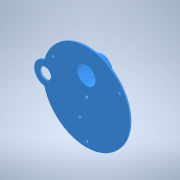
# Autodesk Inventor part: filterTop
Saved by Autodesk Inventor 2022.1 (Build 261234000, 234)
## iProperties
Created: 2020-04-12
Part Number: filterTop
Material: PBT Plastic
Document SubType Name: Modeling
Designer: robst
Density: 1.31 g/cm^3
Appearance: Cyan
Author: robst
Autodesk Inventor part; units mm, degrees
ref_plane "YZ Plane" through (0, 0, 0) normal (1, 0, 0) x (0, 1, 0)
ref_plane "XZ Plane" through (0, 0, 0) normal (0, 1, 0) x (-1, 0, 0)
ref_plane "XY Plane" through (0, 0, 0) normal (0, 0, 1) x (1, 0, 0)
sketch "Sketch7" plane through (0, 0, 0) normal (0, 0, 1) x (1, 0, 0)
  circle A0 centre (0, 0) radius 76.2
  dimension "d15" = 152.4
  constraints: 1 centre point, 1 coincident
  measures "d15" diameter of A0
extrude "Extrusion4" add sketch "Sketch7" against normal blind 2.54
sketch "Sketch8" plane through (0, 0, 0) normal (0, 0, 1) x (1, 0, 0)
  circle A0 centre (0, 33.1656) radius 15.875
  point P0 (0, 0)
  dimension "d18" = 33.1656
  dimension "d19" = 31.75
  constraints: 1 centre point
  measures "d18" distance of A0.centre point (0, 0)
  measures "d19" diameter of A0
extrude "Extrusion5" cut sketch "Sketch8" against normal through all
sketch "Sketch9" plane through (0, 0, -2.54) normal (0, 0, -1) x (-1, 0, 0)
  arc A0 (-49.0406, 0) -> (49.0406, 0) centre (0, 0) ccw construction
  circle A1 centre (0, 33.1656) radius 15.875 construction
  line L0 (49.0406, 0) -> (-49.0406, 0) construction
  line L1 (43.8953, -13.7366) -> (49.0102, -15.3875)
  line L2 (49.0102, -15.3875) -> (49.6384, -13.4412)
  line L3 (49.6384, -13.4412) -> (50.3248, -13.6627)
  line L4 (50.3248, -13.6627) -> (48.8195, -18.3263)
  line L5 (48.8195, -18.3263) -> (48.1332, -18.1048)
  line L6 (48.1332, -18.1048) -> (48.7613, -16.1585)
  line L7 (48.7613, -16.1585) -> (43.6464, -14.5076)
  line L8 (43.6464, -14.5076) -> (43.8953, -13.7366)
  spline S0 degree 2 poles (45.8988, -23.2012) (45.3865, -23.3468) (44.1482, -23.203) (43.4566, -22.8859) knots 0 0 0 1 2 2 2
  spline S1 degree 2 poles (43.4566, -22.8859) (42.783, -22.5771) (41.8482, -21.7356) (41.6282, -21.2435) knots 0 0 0 1 2 2 2
  spline S2 degree 2 poles (41.6282, -21.2435) (41.3985, -20.7251) (41.444, -19.6537) (41.6931, -19.1104) knots 0 0 0 1 2 2 2
  spline S3 degree 2 poles (41.6931, -19.1104) (41.9504, -18.549) (42.7439, -17.8259) (43.2669, -17.6689) knots 0 0 0 1 2 2 2
  spline S4 degree 2 poles (43.2669, -17.6689) (43.7813, -17.5189) (45.02, -17.6737) (45.7026, -17.9866) knots 0 0 0 1 2 2 2
  spline S5 degree 2 poles (45.7026, -17.9866) (46.3986, -18.3057) (47.2999, -19.1373) (47.5354, -19.6312) knots 0 0 0 1 2 2 2
  spline S6 degree 2 poles (47.5354, -19.6312) (47.7554, -20.1233) (47.7234, -21.2009) (47.4681, -21.7577) knots 0 0 0 1 2 2 2
  spline S7 degree 2 poles (47.4681, -21.7577) (47.2087, -22.3236) (46.3977, -23.0495) (45.8988, -23.2012) knots 0 0 0 1 2 2 2
  spline S8 degree 2 poles (43.8086, -22.118) (44.3565, -22.3692) (45.3143, -22.5203) (45.6916, -22.4323) knots 0 0 0 1 2 2 2
  spline S9 degree 2 poles (45.6916, -22.4323) (46.0798, -22.3441) (46.6513, -21.8561) (46.8284, -21.4699) knots 0 0 0 1 2 2 2
  spline S10 degree 2 poles (46.8284, -21.4699) (47.0116, -21.0702) (47.009, -20.3408) (46.8176, -19.976) knots 0 0 0 1 2 2 2
  spline S11 degree 2 poles (46.8176, -19.976) (46.6356, -19.6262) (45.8894, -19.0016) (45.3505, -18.7545) knots 0 0 0 1 2 2 2
  spline S12 degree 2 poles (45.3505, -18.7545) (44.2593, -18.2543) (42.6808, -18.6393) (42.3287, -19.4072) knots 0 0 0 1 2 2 2
  spline S13 degree 2 poles (42.3287, -19.4072) (41.9767, -20.1751) (42.7174, -21.6178) (43.8086, -22.118) knots 0 0 0 1 2 2 2
  spline S14 degree 2 poles (41.8665, -27.8749) (41.5285, -27.6702) (41.0658, -27.0609) (40.985, -26.7174) knots 0 0 0 1 2 2 2
  spline S15 degree 2 poles (40.985, -26.7174) (40.8826, -26.2858) (41.0506, -25.3884) (41.3883, -24.8306) knots 0 0 0 1 2 2 2
  line L9 (41.3883, -24.8306) -> (41.744, -24.2432)
  line L10 (41.744, -24.2432) -> (39.8002, -23.0662)
  line L11 (39.8002, -23.0662) -> (40.2198, -22.3732)
  line L12 (40.2198, -22.3732) -> (45.4343, -25.5307)
  line L13 (45.4343, -25.5307) -> (44.6411, -26.8407)
  spline S16 degree 2 poles (44.6411, -26.8407) (44.3596, -27.3055) (43.8135, -27.8641) (43.4892, -28.0086) knots 0 0 0 1 2 2 2
  spline S17 degree 2 poles (43.4892, -28.0086) (43.1141, -28.1799) (42.3018, -28.1385) (41.8665, -27.8749) knots 0 0 0 1 2 2 2
  spline S18 degree 2 poles (42.2829, -27.1395) (42.5534, -27.3033) (43.0632, -27.3579) (43.3051, -27.2445) knots 0 0 0 1 2 2 2
  spline S19 degree 2 poles (43.3051, -27.2445) (43.5148, -27.1462) (43.8696, -26.7605) (44.0666, -26.4351) knots 0 0 0 1 2 2 2
  line L14 (44.0666, -26.4351) -> (44.4146, -25.8604)
  line L15 (44.4146, -25.8604) -> (42.3356, -24.6015)
  line L16 (42.3356, -24.6015) -> (42.049, -25.0747)
  spline S20 degree 2 poles (42.049, -25.0747) (41.7931, -25.4973) (41.6136, -26.099) (41.6887, -26.3755) knots 0 0 0 1 2 2 2
  spline S21 degree 2 poles (41.6887, -26.3755) (41.7504, -26.6265) (42.0336, -26.9885) (42.2829, -27.1395) knots 0 0 0 1 2 2 2
  constraints: 2 end point, 2 point on circle, 1 centre point, 1 coincident, 1 horizontal, 1 tangent, 1 other
extrude "Extrusion6" cut sketch "Sketch9" against normal blind 0.635
sketch "Sketch10" plane through (0, 0, -2.54) normal (0, 0, -1) x (-1, 0, 0)
  circle A0 centre (0, 33.1656) radius 15.875 projected
  circle A1 centre (0, 33.1656) radius 15.875
  circle A2 centre (0, 33.1656) radius 18.4404
  point P0 (0, 0)
  dimension "d24" = 2.5654
  constraints: 2 centre point, 2 coincident, 1 concentric
  measures "d24" radial gap between concentric circles of A0 A2
extrude "Extrusion7" add sketch "Sketch10" along normal blind 25.4
sketch "Sketch11" plane through (0, 0, -2.54) normal (0, 0, -1) x (-1, 0, 0)
  point P0 (0, 0)
  point P1 (0, 0)
  constraints: 1 coincident
hole "Hole1" at (0, 0, -2.54) direction (0, 0, 1) diameter 5.1054 end through all clearance for "Flat Head Machine Screw (82)" size "#10" standard "Ansi Unified Screw Threads"
sketch "Sketch12" plane through (0, 0, -2.54) normal (0, 0, -1) x (-1, 0, 0)
  circle A0 centre (0, 0) radius 2.5527 construction
  line L0 (0, 0) -> (76.2, 0) construction
  circle A1 centre (0, 0) radius 76.2 construction
  circle A2 centre (0, 0) radius 76.2 construction
  circle A3 centre (71.755, 0) radius 3.175
  dimension "d34" = 6.35
  dimension "d35" = 71.755
  constraints: 2 end point, 2 horizontal alignment, 1 centre point, 1 horizontal, 1 point on line, 1 other
  measures "d34" diameter of A3
  measures "d35" distance of A3.centre point (0, 0)
extrude "Extrusion8" cut sketch "Sketch12" against normal through all
sketch "Sketch13" plane through (0, 0, -2.54) normal (0, 0, -1) x (-1, 0, 0)
  circle A0 centre (0, 0) radius 76.2 projected
  circle A1 centre (71.755, 0) radius 3.175 projected
  arc A2 (74.3072, -16.8785) -> (74.3072, 16.8785) centre (71.755, 0) ccw
  arc A3 (73.658, -19.5178) -> (73.658, 19.5178) centre (71.755, 0) ccw
  circle A4 centre (0, 0) radius 2.5527 projected
  arc A5 (73.658, -19.5178) -> (73.658, 19.5178) centre (0, 0) ccw
  point P0 (76.0567, 4.671)
  point P1 (76.0567, -4.671)
  dimension "d38" = 17.0703
  dimension "d39" = 2.54
  constraints: 10 point on circle, 3 centre point, 3 coincident, 1 concentric, 1 other
  measures "d38" radius of A2
  measures "d39" radial gap between concentric circles of A3 A2
extrude "Extrusion9" add sketch "Sketch13" against normal up to surface (2.54 mm away) contours A0 A2 | A0 A3 A2 | A1
sketch "Sketch14" plane through (0, 0, 0) normal (0, 0, 1) x (1, 0, 0)
  circle A0 centre (0, 0) radius 2.5527 construction
  circle A1 centre (0, 0) radius 38.1 construction
  line L0 (0, 0) -> (0, -38.1) construction
  line L1 (0, 0) -> (-11.7735, -36.2353) construction
  dimension "d42" = 76.2
  dimension "d43" = 18
  constraints: 4 end point, 2 coincident, 2 point on circle, 1 centre point, 1 vertical
  measures "d42" diameter of A1
  measures "d43" angle of L1 L0
hole "Hole2" at (-11.7735, -36.2353, 0) direction (0, 0, -1) diameter 4.4958 end through all clearance for "Flat Head Machine Screw (82)" size "#8" standard "Ansi Unified Screw Threads"
sketch "Sketch15" plane through (0, 0, -2.54) normal (0, 0, -1) x (-1, 0, 0)
  circle A0 centre (0, 0) radius 2.5527 construction
  circle A1 centre (0, 0) radius 67.0077 construction
  line L0 (0, 0) -> (0, 67.0077) construction
  line L1 (0, 0.9037) -> (-57.6351, 34.1794) construction
  point P0 (-0.7826, -67.0032)
  point P1 (58.4178, 32.8238)
  dimension "d51" = 134.0155
  dimension "d52" = 60
  dimension "d55" = 360
  constraints: 4 end point, 2 coincident, 2 point on circle, 1 centre point, 1 point on line, 1 vertical, 4 other
  measures "d51" diameter of A1
  measures "d52" angle of L1 L0
hole "Hole3" at (57.6351, 34.1794, -2.54) at (0.7826, -67.0032, -2.54) at (-58.4178, 32.8238, -2.54) direction (0, 0, 1) diameter 4.4958 end through all clearance for "Flat Head Machine Screw (82)" size "#8" standard "Ansi Unified Screw Threads"
sketch "Sketch16" plane through (0, 0, -2.54) normal (0, 0, -1) x (-1, 0, 0)
  point P0 (0, 0)
  point P1 (71.755, 0)
  dimension "d64" = 71.755
  measures "d64" distance of point (71.755, 0) point (0, 0)
hole "Hole4" at (-71.755, 0, -2.54) direction (0, 0, 1) diameter 19.558 end through all
equation "\"d18\" = radiusForEyepieceHole"
equation "\"d19\" = eyepieceHole"
equation "\"height\" = 31.75"
equation "\"outerDiameter\" = 129.54"
equation "\"outerRadius\" = 0.5 * outerDiameter"
equation "\"centerHoleDiameter\" = 9.525"
equation "\"eyepieceHole\" = 31.75"
equation "\"radiusForEyepieceHole\" = 33.16561"
equation "\"wallThickness\" = 2.54"
body "Solid2"
body "Solid3"
